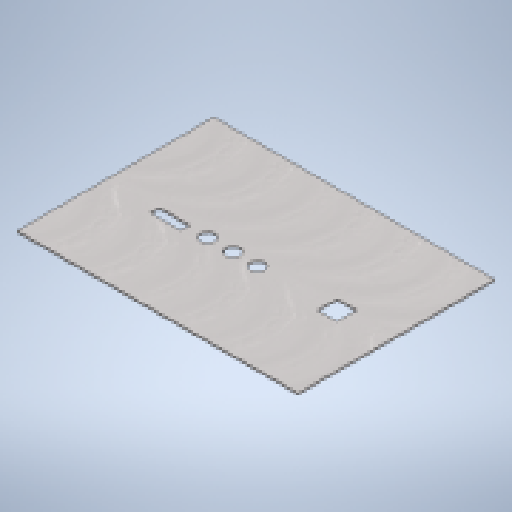
# Autodesk Inventor part: dach
Saved by Autodesk Inventor 2023 (Build 270158000, 158)
## iProperties
Created: 2023-07-07
Part Number: dach
Material: Stal miękka, spawana
Document SubType Name: Modeling
Designer: Kamil
Density: 7.85 g/cm^3
Appearance: Spawane — stal miękka
Author: Kamil
Autodesk Inventor part; units mm, degrees
ref_plane "YZ Plane" through (0, 0, 0) normal (1, 0, 0) x (0, 1, 0)
ref_plane "XZ Plane" through (0, 0, 0) normal (0, 1, 0) x (-1, 0, 0)
ref_plane "XY Plane" through (0, 0, 0) normal (0, 0, 1) x (1, 0, 0)
sketch "Szkic1" plane through (0, 0, 0) normal (0, 1, 0) x (-1, 0, 0)
  line L0 (0, 0) -> (-100, 0)
  line L1 (-100, 0) -> (-100, -70)
  line L2 (-100, -70) -> (0, -70)
  line L3 (0, -70) -> (0, 0)
  dimension "d0" = 100
  dimension "d1" = 70
  constraints: 8 end point, 2 parallel, 1 horizontal, 1 perpendicular
  measures "d0" distance of L2.end L1.end
  measures "d1" distance of L1.end L0.end
extrude "Wyciągnięcie proste1" add sketch "Szkic1" along normal blind 0.5
sketch "Szkic2" plane through (0, 0.5, 0) normal (0, 1, 0) x (1, 0, 0)
  line L0 (84.2801, 35.4995) -> (78.4801, 35.4995) projected
  line L1 (84.3801, 29.5995) -> (84.3801, 35.3995) projected
  line L2 (78.4801, 29.4995) -> (84.2801, 29.4995) projected
  line L3 (78.3801, 35.3995) -> (78.3801, 29.5995) projected
  circle A0 centre (53.6914, 31.8917) radius 2.05 projected
  circle A1 centre (44.8014, 31.8917) radius 2.05 projected
  circle A2 centre (35.9114, 31.8917) radius 2.05 projected
  line L4 (27.6783, 30.5334) -> (27.6783, 31.1734) projected
  line L5 (19.4183, 31.1734) -> (19.4183, 30.5334) projected
  line L6 (84.3801, 29.4995) -> (78.3801, 29.4995)
  line L7 (78.3801, 29.4995) -> (78.3801, 35.4995)
  line L8 (78.3801, 35.4995) -> (84.3801, 35.4995)
  line L9 (84.3801, 35.4995) -> (84.3801, 29.4995)
  line L10 (84.8801, 28.9995) -> (77.8801, 28.9995)
  line L11 (77.8801, 28.9995) -> (77.8801, 35.9995)
  line L12 (77.8801, 35.9995) -> (84.8801, 35.9995)
  line L13 (84.8801, 35.9995) -> (84.8801, 28.9995)
  circle A3 centre (53.6914, 31.8917) radius 2.55
  circle A4 centre (44.8014, 31.8917) radius 2.55
  circle A5 centre (35.9114, 31.8917) radius 2.55
  line L14 (27.6783, 30.5334) -> (19.4183, 30.5334)
  line L15 (19.4183, 30.5334) -> (19.4183, 31.1734)
  line L16 (19.4183, 31.1734) -> (27.6783, 31.1734)
  line L17 (27.6783, 31.1734) -> (27.6783, 30.5334)
  line L18 (28.9783, 32.4734) -> (18.1183, 32.4734)
  line L19 (18.1183, 32.4734) -> (18.1183, 29.2334)
  line L20 (18.1183, 29.2334) -> (28.9783, 29.2334)
  line L21 (28.9783, 29.2334) -> (28.9783, 32.4734)
  point P0 (0, 0)
  dimension "d4" = 0.5
  dimension "d5" = 0.5
  dimension "d6" = 0.5
  dimension "d7" = 0.5
  dimension "d8" = 1.3
  constraints: 32 end point, 8 parallel, 4 perpendicular, 3 centre point, 2 horizontal, 6 other
  measures "d4" distance between parallel lines of L9 L13
  measures "d5" radial gap between concentric circles of A0 A3
  measures "d6" radial gap between concentric circles of A1 A4
  measures "d7" radial gap between concentric circles of A2 A5
  measures "d8" distance between parallel lines of L16 L18
extrude "Wyciągnięcie proste2" cut sketch "Szkic2" against normal through all contours L8 L9 L1 L6 L2 L7 L3 L0 | A0 | A1 | A2 | L14 L5 L16 L4 | L10 L11 L12 L13 | A3 | A4 | A5 | L21 L20 L19 L18
